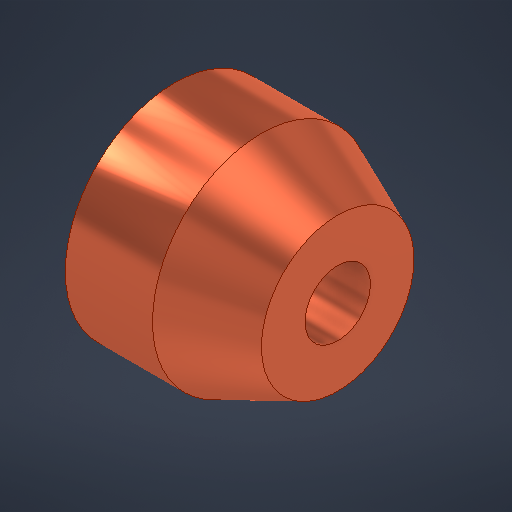
# Autodesk Inventor part: chốt khớp nối
Saved by Autodesk Inventor 2027.1 (Build 311270010, 270A)
## iProperties
Created: 2026-08-09
Part Number: chốt khớp nối
Material: Generic
Document SubType Name: Sheet Metal
Designer: MSI
Density: 1 g/cm^3
Sheet Metal Rule: Default_mm
Appearance: Metal 1400F Hot
Author: MSI
Autodesk Inventor part; units mm, degrees
ref_plane "YZ Plane" through (0, 0, 0) normal (1, 0, 0) x (0, 1, 0)
ref_plane "XZ Plane" through (0, 0, 0) normal (0, 1, 0) x (-1, 0, 0)
ref_plane "XY Plane" through (0, 0, 0) normal (0, 0, 1) x (1, 0, 0)
sketch "Sketch1" plane through (0, 0, 0) normal (0, 0, 1) x (1, 0, 0)
  line L0 (0, 7) -> (4, 7)
  line L1 (0, 3.5) -> (7.5, 3.5)
  line L2 (7.5, 3.5) -> (7.5, 5.5)
  line L3 (7.5, 5.5) -> (4, 7)
  line L4 (0, 2) -> (8.6276, 2)
  line L5 (0, 7) -> (0, 3.5)
  point P0 (0, 0)
  dimension "d0" = 7
  dimension "d1" = 4
  dimension "d3" = 2
  dimension "d4" = 2
  constraints: 12 end point, 1 horizontal, 1 perpendicular, 1 vertical
  measures "d0" distance of point (0, 0) L0.start
  measures "d1" distance of L0.start L0.end
  measures "d3" distance of L1.end L2.end
  measures "d4" distance of point (0, 0) L4.start
revolve "Revolution1" add sketch "Sketch1" angle 360 about axis through (0, 2, 0) along (1, 0, 0)
equation "\"BendRadius\" = Thickness"
equation "\"BendReliefWidth\" = Thickness"
equation "\"BendReliefDepth\" = 0.5 * Thickness"
equation "\"CornerReliefSize\" = 4 * Thickness"
equation "\"MinimumRemnant\" = 2 * Thickness"
equation "\"TransitionRadius\" = BendRadius"
equation "\"JacobiRadiusSize\" = BendRadius"
equation "\"GapSize\" = Thickness"
equation "\"Thickness\" = 0.5"
body "Solid1"
